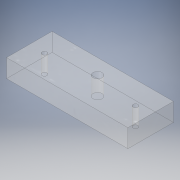
# Autodesk Inventor part: phone_holder_slider_cover
Saved by Autodesk Inventor 2019 (Build 230136000, 136)
## iProperties
Created: 2019-02-17
Part Number: phone_holder_slider_cover
Material: Acrylic, Clear
Document SubType Name: Modeling
Designer: suchanek
Density: 1.19 g/cm^3
Appearance: Transparent - Clear
Author: suchanek
Autodesk Inventor part; units mm, degrees
ref_plane "YZ Plane" through (0, 0, 0) normal (1, 0, 0) x (0, 1, 0)
ref_plane "XZ Plane" through (0, 0, 0) normal (0, 1, 0) x (-1, 0, 0)
ref_plane "XY Plane" through (0, 0, 0) normal (0, 0, 1) x (1, 0, 0)
sketch "Sketch1" plane through (0, 0, 0) normal (0, 1, 0) x (-1, 0, 0)
  line L0 (0, 15) -> (40, 15)
  line L1 (40, 15) -> (40, 0)
  line L2 (40, 0) -> (0, 0)
  line L3 (0, 0) -> (0, 15)
  circle A0 centre (5, 7.5) radius 0.8
  circle A1 centre (35, 7.5) radius 0.8
  circle A2 centre (20, 5) radius 1.5
  dimension "d0" = 1.6
  dimension "d1" = 7.5
  dimension "d2" = 5
  dimension "d3" = 5
  dimension "d4" = 30
  dimension "d8" = 15
  dimension "d9" = 3
  dimension "d10" = 20
  dimension "d11" = 5
  constraints: 8 end point, 3 centre point, 2 parallel, 2 point on line, 1 equal radius, 1 horizontal, 1 horizontal alignment, 1 perpendicular
  measures "d0" diameter of A1
  measures "d1" distance from line of L2 A1.centre
  measures "d2" distance from line of L1 A1.centre
  measures "d3" distance from line of L3 A0.centre
  measures "d4" distance of A0.centre A1.centre
  measures "d8" distance of L0.end L1.end
  measures "d9" diameter of A2
  measures "d10" distance from line of L3 A2.centre
  measures "d11" distance from line of L2 A2.centre
extrude "Extrusion1" add sketch "Sketch1" along normal blind 6
body "Solid1"
